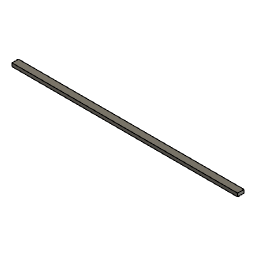
straight (Autodesk Fusion 360 design; units mm, degrees)
Autodesk Fusion 360 part; units mm, degrees
sketch "Sketch1" plane through (0, 0, 0) normal (0, 0, 1) x (1, 0, 0)
  line L0 (0, 0.05) -> (7, 0.05)
  line L1 (7, 0.05) -> (7, -0.05)
  line L2 (7, -0.05) -> (0, -0.05)
  line L3 (0, -0.05) -> (0, 0.05)
  dimension "d27" = 7
  dimension "d28" = 0.1
  constraint horizontal L0
  constraint vertical L1
  constraint horizontal L2
  constraint vertical L3
  constraint midpoint origin L3
  measures "d27" distance of L1.end L2.end
  measures "d28" distance of L0.start L2.end
extrude "Extrude2" add sketch "Sketch1" along normal blind 0.2
equation "d1000 = channelwidth"
equation "d1001 = depth"
equation "channelwidth = 0.1 mm" comment "User edit"
equation "depth = 0.2 mm"
equation "length = 7 mm"
equation "d27 = length"
equation "d28 = channelwidth"
